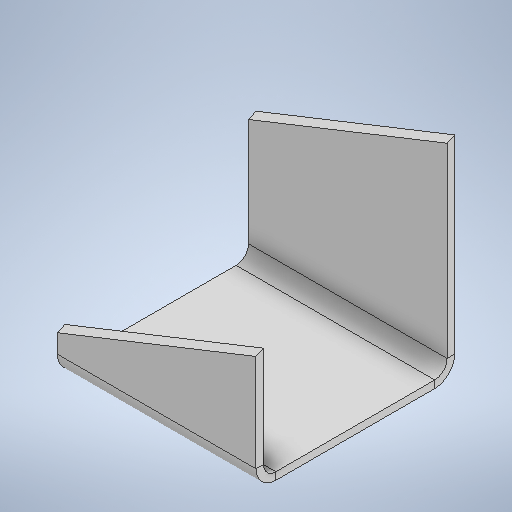
# Autodesk Inventor part: MSC 081 pillar 1
Saved by Autodesk Inventor 2025 (Build 290162010, 162A)
## iProperties
Created: 2024-06-25
Part Number: MSC 081 pillar 1
Material: Stainless Steel
Document SubType Name: Sheet Metal
Designer: admin
Density: 8 g/cm^3
Sheet Metal Rule: AISI304 3mm Die 32
Appearance: Default
Author: admin
Autodesk Inventor part; units mm, degrees
ref_plane "YZ Plane" through (0, 0, 0) normal (1, 0, 0) x (0, 1, 0)
ref_plane "XZ Plane" through (0, 0, 0) normal (0, 1, 0) x (-1, 0, 0)
ref_plane "XY Plane" through (0, 0, 0) normal (0, 0, 1) x (1, 0, 0)
sketch3d "3D Sketch1"
sketch "Sketch1" plane through (0, 0, 0) normal (0, 0, 1) x (1, 0, 0)
  line L0 (-40, 40) -> (40, 40)
  line L1 (40, 40) -> (40, -40)
  line L2 (40, -40) -> (-40, -40)
  line L3 (-40, -40) -> (-40, 40)
  line L4 (-40, 40) -> (40, -40) construction
  line L5 (40, 40) -> (-40, -40) construction
  point P0 (0, 0)
  dimension "d5" = 80
  measures "d5" distance of L1.end L2.end
extrude "Plate1" add sketch "Sketch1" along normal blind 3
sketch "Sketch2" plane through (40, -37, 0) normal (0, -1, 0) x (1, 0, 0)
  line L0 (-80, 0) -> (0, 0)
  line L1 (0, 0) -> (0, 90)
  line L2 (0, 90) -> (-80, 90)
  line L3 (-80, 90) -> (-80, 0)
  constraints: 6 end point, 1 horizontal, 1 perpendicular, 1 vertical
edge flange "Flange1" height 90 angle 90 thickness 3 bend radius 5 thickness toward (0, -1, 0) relief round relief width 3 relief depth 1.5 corner gap 5 corner form 0 edges at (0, -40, 3) (0, 40, 3) wall of the first edge with corners at (-40, -37, 0) (40, -37, 0) (40, -37, 90) (-40, -37, 90)
bend "Bend1"
corner "Corner1"
ref_plane "Work Plane3" through (-34.2655, 0, 36.4126) normal (0.3382043, 0.3977145, -0.8529015) x (0.9295836, 0, 0.3686113)
split "Split1" plane through (-34.2655, 0, 36.4126) removes the side toward (-0.3382043, -0.3977145, 0.8529015)
equation "\"d6\" = Thickness"
equation "\"d7\" = BendReliefWidth"
equation "\"d8\" = BendReliefDepth"
equation "\"d9\" = MinimumRemnant"
equation "\"d10\" = TransitionRadius"
equation "\"d13\" = BendRadius"
equation "\"d14\" = CornerReliefSize"
equation "\"d15\" = GapSize"
equation "\"d16\" = JacobiRadiusSize"
equation "\"BendReliefWidth\" = Thickness"
equation "\"BendReliefDepth\" = 0.5 * Thickness"
equation "\"CornerReliefSize\" = 4 * Thickness"
equation "\"MinimumRemnant\" = 2 * Thickness"
equation "\"TransitionRadius\" = BendRadius"
equation "\"JacobiRadiusSize\" = BendRadius"
equation "\"GapSize\" = Thickness"
equation "\"Thickness\" = 3"
equation "\"BendRadius\" = 5"
body "Solid1"
